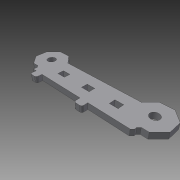
# Autodesk Inventor part: rope_mount_b
Saved by Autodesk Inventor 2014 (Build 180170000, 170)
## iProperties
Created: 2013-12-08
Part Number: rope_mount_b
Material: Generic
Document SubType Name: Modeling
Designer: buben
Density: 1 g/cm^3
Appearance: Default
Author: buben
Autodesk Inventor part; units mm, degrees
ref_plane "YZ Plane" through (0, 0, 0) normal (1, 0, 0) x (0, 1, 0)
ref_plane "XZ Plane" through (0, 0, 0) normal (0, 1, 0) x (-1, 0, 0)
ref_plane "XY Plane" through (0, 0, 0) normal (0, 0, 1) x (1, 0, 0)
sketch "Sketch1" plane through (0, 0, 0) normal (0, 0, 1) x (1, 0, 0)
  circle A0 centre (106.3, 21) radius 13 construction
  circle A1 centre (106.3, 21) radius 17 construction
  circle A2 centre (-2, 21) radius 13 construction
  circle A3 centre (-2, 21) radius 17 construction
  line L0 (-8, 36) -> (112.3, 36)
  line L1 (-8, 36) -> (-17, 27)
  line L2 (-17, 27) -> (-17, 15)
  line L3 (-17, 15) -> (-8, 6)
  circle A4 centre (-2, 21) radius 4.25
  circle A5 centre (106.3, 21) radius 4.25
  line L4 (-8, 6) -> (0, 6)
  line L5 (0, 6) -> (0, 0)
  line L6 (112.3, 36) -> (121.3, 27)
  line L7 (121.3, 27) -> (121.3, 15)
  line L8 (121.3, 15) -> (112.3, 6)
  line L9 (112.3, 6) -> (104.3, 6)
  line L10 (104.3, 6) -> (104.3, 0)
  line L11 (104.3, 0) -> (0, 0)
  point P0 (-17, 21)
  point P1 (-15, 21)
  dimension "d2" = 26
  dimension "d0" = 26
  dimension "d1" = 34
  dimension "d3" = 34
  dimension "d4" = 108.3
  dimension "d5" = 8.5
  dimension "d6" = 8.5
  dimension "d7" = 45
  dimension "d8" = 30
  dimension "d9" = 15
  dimension "d10" = 12
  dimension "d11" = 8
  dimension "d12" = 6
  dimension "d13" = 15
  dimension "d14" = 12
  dimension "d15" = 30
  dimension "d32" = 8
  constraints: 24 end point, 10 perpendicular, 5 centre point, 5 coincident, 4 horizontal alignment, 2 parallel, 1 horizontal, 1 midpoint, 2 other
  measures "d0" diameter of A0
  measures "d1" diameter of A1
  measures "d3" diameter of A3
  measures "d4" distance of A0.centre point (-2, 21)
  measures "d5" diameter of A4
  measures "d6" diameter of A5
  measures "d7" angle of L1 L0
  measures "d8" distance of L3.end L0.start
  measures "d9" distance from line of L2 point (-2, 21)
  measures "d10" distance of L1.end L2.end
  measures "d11" distance of L3.end L4.end
  measures "d12" distance of L4.end L5.end
  measures "d13" distance from line of L7 A0.centre
  measures "d14" distance of L6.end L7.end
  measures "d15" distance from line of L8.end L0
  measures "d32" distance of L8.end L9.end
extrude "Extrusion1" add sketch "Sketch1" along normal blind 6
sketch "Sketch2" plane through (0, 0, 6) normal (0, 0, 1) x (1, 0, 0)
  line L0 (0, 6) -> (0, 0) projected
  line L1 (0, 0) -> (104.3, 0) projected
  line L2 (4, 0) -> (12, 0)
  line L3 (12, 0) -> (12, -4)
  line L4 (10, -6) -> (6, -6)
  line L5 (4, -4) -> (4, 0)
  line L6 (57, 0) -> (65, 0)
  line L7 (65, 0) -> (65, -4)
  line L8 (63, -6) -> (59, -6)
  line L9 (57, -4) -> (57, 0)
  arc A0 (4, -4) -> (6, -6) centre (6, -4) ccw
  arc A1 (10, -6) -> (12, -4) centre (10, -4) ccw
  arc A2 (57, -4) -> (59, -6) centre (59, -4) ccw
  arc A3 (63, -6) -> (65, -4) centre (63, -4) ccw
  dimension "d18" = 2
  dimension "d19" = 8
  dimension "d20" = 8
  dimension "d21" = 6
  dimension "d22" = 4
  dimension "d33" = 45
  constraints: 16 end point, 8 point on circle, 8 tangent, 4 centre point, 4 parallel, 3 equal radius, 2 horizontal, 2 perpendicular, 2 point on line, 1 collinear
  measures "d18" radius of A0
  measures "d19" distance between parallel lines of L3 L5
  measures "d20" distance between parallel lines of L7 L9
  measures "d21" distance between parallel lines of L2 L4
  measures "d22" distance between parallel lines of L0 L5
  measures "d33" distance between parallel lines of L9 L3
extrude "Extrusion2" add sketch "Sketch2" against normal blind 6
sketch "Sketch3" plane through (0, 0, 6) normal (0, 0, 1) x (1, 0, 0)
  line L0 (112.3, 36) -> (-8, 36) projected
  line L1 (121.3, 15) -> (121.3, 27) projected
  line L2 (121.3, 27) -> (112.3, 36) projected
  line L3 (4, 36) -> (13, 27)
  line L4 (13, 27) -> (91.3, 27)
  line L5 (91.3, 27) -> (100.3, 36)
  point P0 (-17, 27)
  point P1 (-17, 15)
  dimension "d26" = 12
  dimension "d27" = 12
  dimension "d28" = 12
  constraints: 6 end point, 2 perpendicular, 2 point on line, 1 horizontal alignment, 1 parallel
  measures "d26" distance of point (-17, 27) point (-17, 15)
  measures "d27" distance of L3.start L0.end
  measures "d28" distance of L0.start L5.end
extrude "Extrusion3" cut sketch "Sketch3" against normal through all
sketch "Sketch4" plane through (0, 0, 6) normal (0, 0, 1) x (1, 0, 0)
  line L0 (12, 0) -> (57, 0) projected
  line L1 (91.3, 27) -> (13, 27) projected
  line L2 (20.15, 16) -> (28.15, 16)
  line L3 (28.15, 16) -> (28.15, 10)
  line L4 (28.15, 10) -> (20.15, 10)
  line L5 (20.15, 10) -> (20.15, 16)
  line L6 (48.15, 16) -> (56.15, 16)
  line L7 (56.15, 16) -> (56.15, 10)
  line L8 (56.15, 10) -> (48.15, 10)
  line L9 (48.15, 10) -> (48.15, 16)
  line L10 (76.15, 16) -> (84.15, 16)
  line L11 (84.15, 16) -> (84.15, 10)
  line L12 (84.15, 10) -> (76.15, 10)
  line L13 (76.15, 10) -> (76.15, 16)
  line L14 (28.15, 13) -> (48.15, 13) construction
  line L15 (56.15, 13) -> (76.15, 13) construction
  point P0 (52.15, 16)
  point P1 (52.15, 27)
  dimension "d34" = 8
  dimension "d35" = 6
  dimension "d36" = 10
  dimension "d37" = 20
  constraints: 28 end point, 7 collinear, 6 midpoint, 6 parallel, 3 horizontal, 3 perpendicular, 1 vertical alignment
  measures "d34" distance of L2.start L2.end
  measures "d35" distance of L4.end L2.start
  measures "d36" distance between parallel lines of L0 L8
  measures "d37" distance of L15.start L15.end
extrude "Extrusion4" cut sketch "Sketch4" against normal through all
chamfer "Chamfer1" distance 2 angle 45 3 edges at (0, 6, 3) (104.3, 6, 3) (104.3, 0, 3)
equation "\"d6\" = d5"
equation "\"d27\" = d26"
equation "\"d28\" = d26"
body "Solid1"
